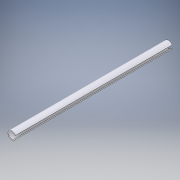
# Autodesk Inventor part: inner_sheath
Saved by Autodesk Inventor 2017 (Build 210142000, 142)
## iProperties
Created: 2018-11-30
Part Number: inner_sheath
Material: Acetal Resin, White
Document SubType Name: Modeling
Designer: ddeboer
Density: 1.425 g/cm^3
Appearance: Smooth - White
Author: ddeboer
Autodesk Inventor part; units mm, degrees
ref_plane "YZ Plane" through (0, 0, 0) normal (1, 0, 0) x (0, 1, 0)
ref_plane "XZ Plane" through (0, 0, 0) normal (0, 1, 0) x (-1, 0, 0)
ref_plane "XY Plane" through (0, 0, 0) normal (0, 0, 1) x (1, 0, 0)
sketch "Sketch1" plane through (0, 0, 0) normal (0, 0, 1) x (1, 0, 0)
  circle A0 centre (0, 0) radius 13.27
  circle A1 centre (0, 0) radius 10.325
  dimension "d0" = 26.54
  dimension "d1" = 20.65
  constraints: 2 centre point, 2 coincident
  measures "d0" diameter of A0
  measures "d1" diameter of A1
extrude "Extrusion1" add sketch "Sketch1" along normal blind 520
sketch "Sketch4" plane through (0, 0, 0) normal (0, 0, -1) x (-1, 0, 0)
  line L0 (-20, 5.75) -> (0, 5.75)
  line L1 (0, 5.75) -> (0, -5.75)
  line L2 (0, -5.75) -> (-20, -5.75)
  line L3 (-20, -5.75) -> (-20, 5.75)
  point P0 (0, 0)
  point P1 (0, 0)
  dimension "d9" = 20
  dimension "d10" = 11.5
  constraints: 8 end point, 2 parallel, 1 coincident, 1 horizontal, 1 midpoint, 1 perpendicular
  measures "d9" distance of L1.end L2.end
  measures "d10" distance of L0.end L1.end
extrude "Extrusion4" cut sketch "Sketch4" against normal up to next
body "Solid1"
